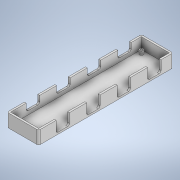
# Autodesk Inventor part: Box
Saved by Autodesk Inventor 2021 (Build 250183000, 183)
## iProperties
Created: 2023-03-09
Part Number: Box
Material: Generic
Document SubType Name: Modeling
Designer: mathe
Density: 1 g/cm^3
Appearance: Default
Author: mathe
Autodesk Inventor part; units mm, degrees
ref_plane "YZ Plane" through (0, 0, 0) normal (1, 0, 0) x (0, 1, 0)
ref_plane "XZ Plane" through (0, 0, 0) normal (0, 1, 0) x (-1, 0, 0)
ref_plane "XY Plane" through (0, 0, 0) normal (0, 0, 1) x (1, 0, 0)
sketch "Sketch1" plane through (0, 0, 0) normal (0, 1, 0) x (-1, 0, 0)
  line L0 (0, 0) -> (35.179, 0)
  line L1 (35.179, 0) -> (35.179, -210.947)
  line L2 (35.179, -210.947) -> (0, -210.947)
  line L3 (0, -210.947) -> (0, 0)
  circle A0 centre (35.179, 0) radius 1.45
  circle A1 centre (0, 0) radius 1.45
  circle A2 centre (35.179, -210.947) radius 1.45
  line L4 (-6.35, 6.35) -> (41.529, 6.35)
  line L5 (41.529, 6.35) -> (41.529, -217.297)
  line L6 (41.529, -217.297) -> (-6.35, -217.297)
  line L7 (-6.35, -217.297) -> (-6.35, 6.35)
  line L8 (-6.35, 6.35) -> (41.529, -217.297) construction
  line L9 (41.529, 6.35) -> (-6.35, -217.297) construction
  line L10 (28.829, -204.597) -> (41.529, -204.597)
  line L11 (41.529, -204.597) -> (41.529, -217.297)
  line L12 (41.529, -217.297) -> (28.829, -217.297)
  line L13 (28.829, -217.297) -> (28.829, -204.597)
  line L14 (28.829, -204.597) -> (41.529, -217.297) construction
  line L15 (41.529, -204.597) -> (28.829, -217.297) construction
  line L16 (-9.525, 9.525) -> (44.704, 9.525)
  line L17 (44.704, 9.525) -> (44.704, -220.472)
  line L18 (44.704, -220.472) -> (-9.525, -220.472)
  line L19 (-9.525, -220.472) -> (-9.525, 9.525)
  line L20 (-9.525, 9.525) -> (44.704, -220.472) construction
  line L21 (44.704, 9.525) -> (-9.525, -220.472) construction
  point P0 (17.5895, -105.4735)
  point P1 (17.5895, -105.4735)
  dimension "d0" = 35.179
  dimension "d1" = 210.947
  dimension "d2" = 2.9
  dimension "d3" = 2.9
  dimension "d4" = 2.9
  dimension "d6" = 12.7
  dimension "d7" = 12.7
  dimension "d8" = 3.175
  dimension "d9" = 3.175
  constraints: 44 end point, 8 parallel, 7 midpoint, 4 horizontal, 4 perpendicular, 3 centre point, 3 coincident, 1 other
  measures "d0" distance of L1.end L2.end
  measures "d1" distance of L0.end L1.end
  measures "d2" diameter of A0
  measures "d3" diameter of A1
  measures "d4" diameter of A2
  measures "d6" distance of L12.end L10.start
  measures "d7" distance of L10.start L10.end
  measures "d8" distance between parallel lines of L5 L17
  measures "d9" distance between parallel lines of L18 L6
extrude "Extrusion1" add sketch "Sketch1" along normal blind 3.175 contours A1 L3 L2 L13 L6 L7 L4 L5 L10 L1 A0 L0 | L0 A0 L1 L10 L13 L2 L3 A1 | L13 L10 L1 A2 L2 | L2 A2 L1 L10 L5 L6 L13 | L16 L17 L18 L19
extrude "Extrusion2" add sketch "Sketch1" along normal blind 22.225
sketch "Sketch2" plane through (0, 3.175, 0) normal (0, 1, 0) x (1, 0, 0)
  circle A0 centre (-35.1446, 0) radius 3.175
  circle A1 centre (0, 0) radius 3.175
  circle A2 centre (-35.179, 0) radius 1.45 projected
  circle A3 centre (0, 0) radius 1.45 projected
  circle A4 centre (-35.179, 210.947) radius 1.45 projected
  circle A5 centre (-35.179, 210.947) radius 3.175
  point P0 (0, 210.947)
  dimension "d14" = 6.35
  dimension "d15" = 6.35
  dimension "d20" = 6.35
  constraints: 3 centre point, 2 coincident
  measures "d14" diameter of A0
  measures "d15" diameter of A1
  measures "d20" diameter of A5
extrude "Extrusion3" add sketch "Sketch2" along normal blind 6.35
extrude "Extrusion4" add sketch "Sketch1" along normal blind 3.175 contours L3 A1 L0 | L0 A1 L3 | A0 L1 L0 | L0 L1 A0 | A2 L1 L2 | L2 L1 A2
sketch "Sketch3" plane through (0, 22.225, 0) normal (0, 1, 0) x (1, 0, 0)
  circle A0 centre (-25.011, 12.319) radius 6.5
  circle A1 centre (-25.011, 50.292) radius 6.5
  circle A2 centre (-25.011, 64.516) radius 6.5
  circle A3 centre (-25.011, 102.489) radius 6.5
  circle A4 centre (-25.011, 116.713) radius 6.5
  circle A5 centre (-25.011, 154.686) radius 6.5
  circle A6 centre (-25.011, 168.91) radius 6.5
  circle A7 centre (-25.011, 206.883) radius 6.5
  line L0 (-9.707, 199.896) -> (-9.707, 209.896)
  line L1 (-9.707, 209.896) -> (2.293, 209.896)
  line L2 (2.293, 209.896) -> (2.293, 199.896)
  line L3 (2.293, 199.896) -> (-9.707, 199.896)
  line L4 (-9.707, 177.003) -> (2.293, 177.003)
  line L5 (-9.707, 167.003) -> (-9.707, 177.003)
  line L6 (2.293, 167.003) -> (-9.707, 167.003)
  line L7 (2.293, 177.003) -> (2.293, 167.003)
  line L8 (2.293, 157.699) -> (2.293, 147.699)
  line L9 (-9.707, 157.699) -> (2.293, 157.699)
  line L10 (2.293, 147.699) -> (-9.707, 147.699)
  line L11 (-9.707, 147.699) -> (-9.707, 157.699)
  line L12 (-9.707, 124.806) -> (2.293, 124.806)
  line L13 (-9.707, 114.806) -> (-9.707, 124.806)
  line L14 (2.293, 114.806) -> (-9.707, 114.806)
  line L15 (2.293, 124.806) -> (2.293, 114.806)
  line L16 (-9.707, 105.502) -> (2.293, 105.502)
  line L17 (2.293, 105.502) -> (2.293, 95.502)
  line L18 (-9.707, 95.502) -> (-9.707, 105.502)
  line L19 (2.293, 95.502) -> (-9.707, 95.502)
  line L20 (-9.707, 72.609) -> (2.293, 72.609)
  line L21 (-9.707, 62.609) -> (-9.707, 72.609)
  line L22 (2.293, 62.609) -> (-9.707, 62.609)
  line L23 (2.293, 72.609) -> (2.293, 62.609)
  line L24 (-9.707, 53.305) -> (2.293, 53.305)
  line L25 (-9.707, 43.305) -> (-9.707, 53.305)
  line L26 (2.293, 43.305) -> (-9.707, 43.305)
  line L27 (2.293, 53.305) -> (2.293, 43.305)
  line L28 (-9.707, 20.412) -> (2.293, 20.412)
  line L29 (2.293, 20.412) -> (2.293, 10.412)
  line L30 (2.293, 10.412) -> (-9.707, 10.412)
  line L31 (-9.707, 10.412) -> (-9.707, 20.412)
  line L32 (-17.686, -1.671) -> (-20.286, -1.671)
  line L33 (-23.811, 2.214) -> (-23.811, 0.214)
  line L34 (-14.161, 2.214) -> (-14.161, 0.214)
  line L35 (-18.511, 3.894) -> (-17.511, 3.894)
  line L36 (-20.461, 3.894) -> (-19.461, 3.894)
  line L37 (-35.859, 30.096) -> (-35.859, 20.096)
  line L38 (-35.859, 42.669) -> (-35.859, 32.669)
  line L39 (-35.859, 82.293) -> (-35.859, 72.293)
  line L40 (-35.859, 94.866) -> (-35.859, 84.866)
  line L41 (-35.859, 134.49) -> (-35.859, 124.49)
  line L42 (-35.859, 147.063) -> (-35.859, 137.063)
  line L43 (-35.859, 186.687) -> (-35.859, 176.687)
  line L44 (-35.859, 199.26) -> (-35.859, 189.26)
  line L45 (-17.0795, 187.3678) -> (-17.0795, 189.3599)
  line L46 (-13.5395, 185.2639) -> (-17.0795, 185.2639)
  line L47 (-17.0795, 191.4639) -> (-13.5395, 191.4639)
  line L48 (-13.5395, 191.4639) -> (-13.5395, 185.2639)
  line L49 (-13.5395, 139.2668) -> (-13.5395, 133.0668)
  line L50 (-17.0795, 139.2668) -> (-13.5395, 139.2668)
  line L51 (-17.0795, 135.1708) -> (-17.0795, 137.1629)
  line L52 (-13.5395, 133.0668) -> (-17.0795, 133.0668)
  line L53 (-13.5395, 87.0699) -> (-13.5395, 80.8699)
  line L54 (-13.5395, 80.8699) -> (-17.0795, 80.8699)
  line L55 (-17.0795, 87.0699) -> (-13.5395, 87.0699)
  line L56 (-17.0795, 82.9738) -> (-17.0795, 84.9659)
  line L57 (-17.0795, 30.7768) -> (-17.0795, 32.7689)
  line L58 (-13.5395, 28.6728) -> (-17.0795, 28.6728)
  line L59 (-17.0795, 34.8728) -> (-13.5395, 34.8728)
  line L60 (-13.5395, 34.8728) -> (-13.5395, 28.6728)
  line L61 (3.1921, 139.1709) -> (3.1921, 133.1709)
  line L62 (3.1921, 86.9739) -> (3.1921, 80.9739)
  line L63 (3.1921, 34.7769) -> (3.1921, 28.7769)
  line L64 (3.1921, 191.3679) -> (3.1921, 185.3679)
  circle A8 centre (-35.179, 0) radius 1.702
  circle A9 centre (0, 0) radius 1.702
  circle A10 centre (-35.179, 210.947) radius 1.702
  line L65 (9.525, 220.472) -> (-44.704, 220.472) projected
  line L66 (-44.704, 220.472) -> (-44.704, -9.525) projected
  line L67 (-44.704, -9.525) -> (9.525, -9.525) projected
  line L68 (9.525, -9.525) -> (9.525, 220.472) projected
  line L69 (6.35, -6.35) -> (-41.529, -6.35) projected
  line L70 (-41.529, -6.35) -> (-41.529, 217.297) projected
  line L71 (-41.529, 217.297) -> (6.35, 217.297) projected
  line L72 (6.35, 217.297) -> (6.35, -6.35) projected
  line L73 (9.525, -9.525) -> (9.525, 220.472) projected
  line L74 (6.35, 20.412) -> (9.525, 20.412)
  line L75 (9.525, 20.412) -> (9.525, 43.305)
  line L76 (9.525, 43.305) -> (6.35, 43.305)
  line L77 (6.35, 43.305) -> (6.35, 20.412)
  line L78 (6.35, 217.297) -> (6.35, -6.35) projected
  line L79 (6.35, 72.609) -> (9.525, 72.609)
  line L80 (9.525, 72.609) -> (9.525, 95.502)
  line L81 (9.525, 95.502) -> (6.35, 95.502)
  line L82 (6.35, 95.502) -> (6.35, 72.609)
  line L83 (6.35, 124.806) -> (9.525, 124.806)
  line L84 (9.525, 124.806) -> (9.525, 147.699)
  line L85 (9.525, 147.699) -> (6.35, 147.699)
  line L86 (6.35, 147.699) -> (6.35, 124.806)
  line L87 (6.35, 177.003) -> (9.525, 177.003)
  line L88 (9.525, 177.003) -> (9.525, 199.896)
  line L89 (9.525, 199.896) -> (6.35, 199.896)
  line L90 (6.35, 199.896) -> (6.35, 177.003)
  line L91 (-41.529, 217.297) -> (-41.529, -6.35) projected
  line L92 (-44.704, 220.472) -> (-44.704, -9.525) projected
  line L93 (-41.529, 20.412) -> (-44.704, 20.412)
  line L94 (-44.704, 20.412) -> (-44.704, 43.305)
  line L95 (-44.704, 43.305) -> (-41.529, 43.305)
  line L96 (-41.529, 43.305) -> (-41.529, 20.412)
  line L97 (-41.529, 72.293) -> (-44.704, 72.293)
  line L98 (-44.704, 72.293) -> (-44.704, 95.502)
  line L99 (-44.704, 95.502) -> (-41.529, 95.502)
  line L100 (-41.529, 95.502) -> (-41.529, 72.293)
  line L101 (-41.529, 124.806) -> (-44.704, 124.806)
  line L102 (-44.704, 124.806) -> (-44.704, 147.699)
  line L103 (-44.704, 147.699) -> (-41.529, 147.699)
  line L104 (-41.529, 147.699) -> (-41.529, 124.806)
  line L105 (-41.529, 177.003) -> (-44.704, 177.003)
  line L106 (-44.704, 177.003) -> (-44.704, 199.896)
  line L107 (-44.704, 199.896) -> (-41.529, 199.896)
  line L108 (-41.529, 199.896) -> (-41.529, 177.003)
  point P0 (0, 0)
  constraints: 194 end point, 23 point on line, 16 parallel, 11 centre point, 8 horizontal, 8 perpendicular
extrude "Extrusion5" cut sketch "Sketch3" against normal blind 12.7 contours L107 L70 L105 L66 | L103 L70 L101 L66 | L99 L70 L97 L66 | L95 L70 L93 L66
extrude "Extrusion6" cut sketch "Sketch3" against normal up to surface (19.05 mm away) contours L68 L87 L72 L89 | L68 L83 L72 L85 | L68 L79 L72 L81 | L68 L74 L72 L76
fillet "Fillet1" radius 3.175 16 edges at (7.9375, 3.175, -20.412) (7.9375, 3.175, -43.305) (7.9375, 3.175, -72.609) (7.9375, 3.175, -95.502) (7.9375, 3.175, -124.806) (7.9375, 3.175, -147.699) (7.9375, 3.175, -199.896) (7.9375, 3.175, -177.003) (-43.1165, 9.525, -20.412) (-43.1165, 9.525, -43.305) (-43.1165, 9.525, -95.502) (-43.1165, 9.525, -147.699) (-43.1165, 9.525, -199.896) (-43.1165, 9.525, -72.293) (-43.1165, 9.525, -124.806) (-43.1165, 9.525, -177.003)
fillet "Fillet2" radius 3.175 4 edges at (9.525, 11.1125, 9.525) (9.525, 11.1125, -220.472) (-44.704, 11.1125, -220.472) (-44.704, 11.1125, 9.525)
body "Solid1"
